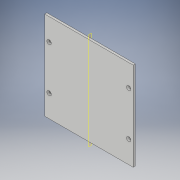
# Autodesk Inventor part: wheel coreBack
Saved by Autodesk Inventor 2018 (Build 220112000, 112)
## iProperties
Created: 2018-08-07
Part Number: wheel coreBack
Material: Generic
Document SubType Name: Modeling
Designer: Cole Tucker
Density: 1 g/cm^3
Appearance: Default
Author: Cole Tucker
Autodesk Inventor part; units mm, degrees
ref_plane "YZ Plane" through (0, 0, 0) normal (1, 0, 0) x (0, 1, 0)
ref_plane "XZ Plane" through (0, 0, 0) normal (0, 1, 0) x (-1, 0, 0)
ref_plane "XY Plane" through (0, 0, 0) normal (0, 0, 1) x (1, 0, 0)
sketch "Sketch1" plane through (0, 0, 0) normal (0, 0, 1) x (1, 0, 0)
  line L0 (0, 0) -> (127, 0)
  line L1 (127, 0) -> (127, 127)
  line L2 (127, 127) -> (0, 127)
  line L3 (0, 127) -> (0, 0)
  dimension "d0" = 127
  dimension "d1" = 127
  constraints: 8 end point, 2 parallel, 1 horizontal, 1 perpendicular
  measures "d0" distance of L2.end L1.end
  measures "d1" distance of L1.end L0.end
extrude "Extrusion1" add sketch "Sketch1" along normal blind 3.175
sketch "Sketch2" plane through (0, 0, 3.175) normal (0, 0, 1) x (1, 0, 0)
  line L0 (127, 127) -> (0, 127) construction
  line L1 (0, 127) -> (0, 101.6) construction
  line L2 (0, 127) -> (0, 0) construction
  line L3 (0, 0) -> (127, 0) construction
  line L4 (0, 0) -> (0, 25.4) construction
  line L5 (0, 25.4) -> (6.35, 25.4) construction
  line L6 (6.35, 25.4) -> (6.35, 31.75) construction
  line L7 (6.35, 31.75) -> (0, 31.75) construction
  line L8 (0, 31.75) -> (0, 25.4) construction
  line L9 (0, 101.6) -> (6.35, 101.6) construction
  line L10 (6.35, 101.6) -> (6.35, 95.25) construction
  line L11 (6.35, 95.25) -> (0, 95.25) construction
  line L12 (0, 95.25) -> (0, 101.6) construction
  dimension "d4" = 25.4
  dimension "d5" = 25.4
  dimension "d6" = 6.35
  dimension "d7" = 6.35
  dimension "d8" = 6.35
  dimension "d9" = 6.35
  constraints: 20 end point, 4 parallel, 2 coincident, 2 horizontal, 2 perpendicular, 2 point on line
  measures "d4" distance of L0.end L1.end
  measures "d5" distance of L2.end L4.end
  measures "d6" distance of L7.end L6.end
  measures "d7" distance of L6.end L5.end
  measures "d8" distance of L10.end L11.end
  measures "d9" distance of L9.end L10.end
ref_plane "Work Plane1" through (63.5, 0, 0) normal (1, 0, 0) x (0, 0, -1)
hole "Hole1" at (6.35, 95.25, 3.175) at (6.35, 31.75, 3.175) direction (0, 0, -1) diameter 3.175 depth 25.4 tip angle 118 countersink diameter 6.35 countersink angle 82
mirror "Mirror1" about plane through (63.5, 0, 0) normal (1, 0, 0) of "Hole1"
body "Solid1"
